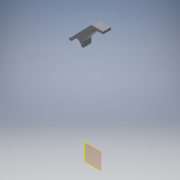
# Autodesk Inventor part: Lin_gage
Saved by Autodesk Inventor 2019.3 (Build 233278000, 278)
## iProperties
Created: 2020-09-17
Part Number: Lin_gage
Material: Generisch
Document SubType Name: Modeling
Designer: Nicolas Frick
Density: 1 g/cm^3
Appearance: Vorgabe
Author: Nicolas Frick
Autodesk Inventor part; units mm, degrees
ref_plane "YZ Plane" through (0, 0, 0) normal (1, 0, 0) x (0, 1, 0)
ref_plane "XZ Plane" through (0, 0, 0) normal (0, 1, 0) x (-1, 0, 0)
ref_plane "XY Plane" through (0, 0, 0) normal (0, 0, 1) x (1, 0, 0)
ref_plane "Arbeitsebene3" through (0, 0, 0) normal (0, 0, 1) x (1, 0, 0)
sketch "Skizze1" plane through (0, 0, 0) normal (0, 0, 1) x (1, 0, 0)
  circle A0 centre (871.1765, 73.7926) radius 2.6 construction
  circle A1 centre (881.1765, 21.442) radius 2.6 construction
  circle A2 centre (28.8235, 21.442) radius 2.6 construction
  circle A3 centre (38.8235, 73.7926) radius 2.6 construction
  line L0 (910, 0) -> (0, 0) construction
  line L1 (910, 0) -> (910, 139) construction
  line L2 (0, 139) -> (910, 139) construction
  line L3 (0, 0) -> (0, 139) construction
  circle A4 centre (-21.0024, 109.9626) radius 6 construction
  line L4 (0, 134.7877) -> (0, 139)
  line L5 (0, 141.9626) -> (-2.1715, 141.9626)
  line L6 (12.5314, 139) -> (0, 139)
  line L7 (0, 141.9626) -> (12.5314, 141.9626)
  line L8 (12.5314, 141.9626) -> (12.5314, 139)
  line L9 (-12.3384, 111.9626) -> (-12.3384, 119.1463)
  line L10 (-12.3384, 119.1463) -> (0, 134.7877)
  line L11 (-21.0024, 109.9626) -> (-21.0024, 111.9626) construction
  arc A5 (-14.8524, 111.9626) -> (-27.1524, 111.9626) centre (-21.0024, 111.9626) ccw
  line L12 (-30.2709, 111.9626) -> (-30.2709, 113.0226)
  line L13 (-30.2709, 113.0226) -> (-2.1715, 141.9626)
  arc A6 (-27.0706, 110.9626) -> (-27.1524, 111.9626) centre (-21.0024, 111.9626) ccw construction
  line L14 (-27.1524, 111.9626) -> (-30.2709, 111.9626)
  line L15 (-14.8524, 111.9626) -> (-12.3384, 111.9626)
  constraints: 24 end point, 5 point on circle, 3 coincident, 3 point on line, 3 vertical, 2 centre point, 1 horizontal, 1 parallel, 1 perpendicular
extrude "Extrusion1" add sketch "Skizze1" against normal blind 10
